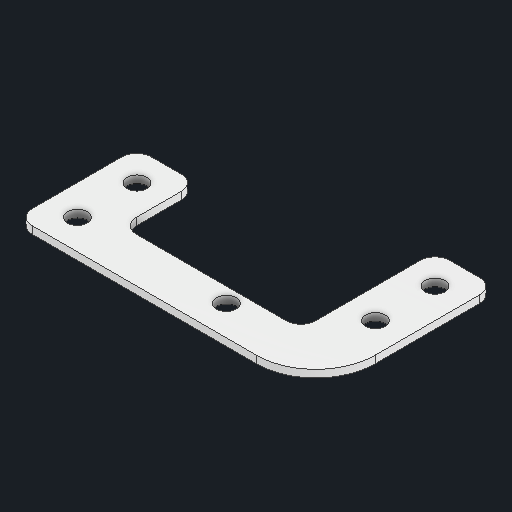
# Autodesk Inventor part: MOGO Funnel
Saved by Autodesk Inventor 2025 (Build 290162000, 162)
## iProperties
Created: 2024-12-27
Part Number: MOGO Funnel
Material: Acetal Resin, White
Document SubType Name: Sheet Metal
Designer: Averey Ku
Density: 1.425 g/cm^3
Appearance: Smooth - White
Flat Pattern Width: 6.35879 cm
Flat Pattern Length: 3.81 cm
Flat Pattern Area: 24.227 cm^2
Sheet Metal Rule: Default_mm
Sheet Metal Width: 2.503 in
Sheet Metal Length: 1.500 in
Sheet Metal Area: 3.755 in^2
Mass: 3.54322 g
Surface Area: 36.7606 cm^2
Volume: 2.48647 cm^3
Author: Averey Ku
Autodesk Inventor part; units mm, degrees
ref_plane "YZ Plane" through (0, 0, 0) normal (1, 0, 0) x (0, 1, 0)
ref_plane "XZ Plane" through (0, 0, 0) normal (0, 1, 0) x (-1, 0, 0)
ref_plane "XY Plane" through (0, 0, 0) normal (0, 0, 1) x (1, 0, 0)
sketch "main" plane through (0, 0, 0) normal (0, 0, 1) x (1, 0, 0)
  point P0 (-4.8343, 8.0815)
sketch "Sketch1" plane through (0, 0, 0) normal (0, 1, 0) x (-1, 0, 0)
  circle A0 centre (0, 0) radius 2.0955
  circle A1 centre (0, 12.7) radius 2.0955
  circle A2 centre (-50.8, 0) radius 2.0955
  line L0 (6.4379, -3.175) -> (6.4379, 15.875)
  line L1 (3.2629, 19.05) -> (-6.2621, 19.05)
  line L2 (-6.2621, 6.35) -> (-6.2621, -3.175)
  line L3 (-3.0871, -6.35) -> (3.2629, -6.35)
  line L4 (-6.2621, 19.05) -> (-44.45, 19.05)
  line L5 (-44.45, -15.875) -> (-44.45, 6.35)
  line L6 (-9.4371, 9.525) -> (-41.275, 9.525)
  line L7 (-57.15, 6.35) -> (-57.15, -15.875)
  line L8 (-53.975, -19.05) -> (-47.625, -19.05)
  arc A3 (-44.45, 19.05) -> (-57.15, 6.35) centre (-44.45, 6.35) ccw
  arc A4 (3.2629, -6.35) -> (6.4379, -3.175) centre (3.2629, -3.175) ccw
  arc A5 (-6.2621, -3.175) -> (-3.0871, -6.35) centre (-3.0871, -3.175) ccw
  arc A6 (6.4379, 15.875) -> (3.2629, 19.05) centre (3.2629, 15.875) ccw
  arc A7 (-47.625, -19.05) -> (-44.45, -15.875) centre (-47.625, -15.875) ccw
  arc A8 (-57.15, -15.875) -> (-53.975, -19.05) centre (-53.975, -15.875) ccw
  arc A9 (-6.2621, 6.35) -> (-9.4371, 9.525) centre (-9.4371, 6.35) ccw
  arc A10 (-41.275, 9.525) -> (-44.45, 6.35) centre (-41.275, 6.35) ccw
  circle A11 centre (-31.75, 12.7) radius 2.0955
  circle A12 centre (-50.8, -12.7) radius 2.0955
  point P0 (-44.45, -19.05)
  point P1 (-57.15, -19.05)
  point P2 (-50.8, -19.05)
  dimension "d17" = 4.191
  dimension "d19" = 12.7
  dimension "d20" = 3.175
  dimension "d21" = 3.175
  dimension "d22" = 4.191
  dimension "d23" = 6.35
  constraints: 18 end point, 16 point on circle, 16 tangent, 13 centre point, 5 equal radius, 4 parallel, 4 point on line, 3 horizontal, 3 vertical, 2 perpendicular, 1 coincident, 1 midpoint, 1 other
  measures "d17" diameter of A0
  measures "d19" distance of point (-57.15, -19.05) point (-44.45, -19.05)
  measures "d20" radius of A4
  measures "d21" radius of A9
  measures "d22" diameter of A11
  measures "d23" distance of point (-50.8, -19.05) A12.centre
extrude "Extrusion1" add sketch "Sketch1" along normal blind 1.5875
equation "\"BendRadius\" = Thickness"
equation "\"BendReliefWidth\" = Thickness"
equation "\"BendReliefDepth\" = 0.5 * Thickness"
equation "\"CornerReliefSize\" = 4 * Thickness"
equation "\"MinimumRemnant\" = 2 * Thickness"
equation "\"TransitionRadius\" = BendRadius"
equation "\"JacobiRadiusSize\" = BendRadius"
equation "\"GapSize\" = Thickness"
equation "\"Thickness\" = 1.5875"
body "Solid1"
